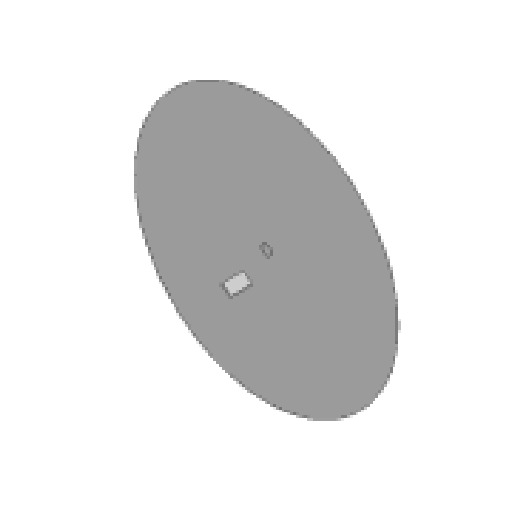
# Autodesk Inventor part: world
Saved by Autodesk Inventor 2023 (Build 270158000, 158)
## iProperties
Created: 2022-08-15
Part Number: world
Material: Generic
Document SubType Name: Modeling
Designer: Derm
Density: 1 g/cm^3
Appearance: Default
Author: Derm
Autodesk Inventor part; units mm, degrees
ref_plane "YZ Plane" through (0, 0, 0) normal (1, 0, 0) x (0, 1, 0)
ref_plane "XZ Plane" through (0, 0, 0) normal (0, 1, 0) x (-1, 0, 0)
ref_plane "XY Plane" through (0, 0, 0) normal (0, 0, 1) x (1, 0, 0)
sketch "Sketch1" plane through (0, 0, 0) normal (0, 0, 1) x (1, 0, 0)
  circle A0 centre (0, 0) radius 12500
  dimension "d8" = 25000
  constraints: 1 centre point, 1 coincident
  measures "d8" diameter of A0
extrude "Extrusion1" add sketch "Sketch1" against normal blind 25.4
sketch "Sketch2" plane through (0, 0, 0) normal (0, 0, 1) x (1, 0, 0)
  circle A0 centre (0, 0) radius 12500 projected
  circle A1 centre (0, 0) radius 500
  circle A2 centre (0, 0) radius 474.6
  dimension "d2" = 1000
  dimension "d7" = 25.4
  constraints: 2 centre point, 1 coincident
  measures "d2" diameter of A1
  measures "d7" radial gap between concentric circles of A1 A2
extrude "Extrusion2" cut sketch "Sketch2" against normal blind 0.254 contours A1
sketch "Sketch3" plane through (0, 0, 0) normal (0, 0, 1) x (1, 0, 0)
  circle A0 centre (0, 0) radius 500 projected
  circle A1 centre (0, 0) radius 12500 projected
  circle A2 centre (0, 0) radius 500 projected
  line L0 (4523.4478, -4083.8637) -> (3719.9636, -4724.5165)
  line L1 (3719.9636, -4724.5165) -> (3734.5609, -4742.824)
  line L2 (3734.5609, -4742.824) -> (4538.0452, -4102.1712)
  line L3 (4538.0452, -4102.1712) -> (4523.4478, -4083.8637)
  line L4 (4523.4478, -4083.8637) -> (3734.5609, -4742.824) construction
  line L5 (3719.9636, -4724.5165) -> (4538.0452, -4102.1712) construction
  line L6 (-652.5808, -3013.9209) -> (-1932.2093, -2136.7742)
  line L7 (-1932.2093, -2136.7742) -> (-1840.266, -2002.6424)
  line L8 (-1840.266, -2002.6424) -> (-560.6375, -2879.7891)
  line L9 (-560.6375, -2879.7891) -> (-652.5808, -3013.9209)
  point P0 (4129.0044, -4413.3439)
  point P1 (-1564.9759, -4707.8399)
  constraints: 20 end point, 4 parallel, 2 midpoint, 2 perpendicular
extrude "Extrusion3" add sketch "Sketch3" along normal blind 2000 contours L6 L7 L8 L9
sketch "Sketch4" plane through (-560.6375, -2879.7891, 0) normal (0.5653912, 0.8248229, 0) x (0.8248229, -0.5653912, 0)
  line L0 (-1551.3979, 0) -> (0, 0) projected
  line L1 (0, 0) -> (0, -2000) projected
  line L2 (0, -2000) -> (-1551.3979, -2000) projected
  line L3 (-1551.3979, 0) -> (-1551.3979, -2000) projected
  point P0 (-1165.7807, 0)
extrude "Extrusion4" add sketch "Sketch4" along normal blind 200
body "Solid1"
